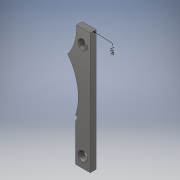
# Autodesk Inventor part: 1-4inch_FixedKnifeSmall_Piece1
Saved by Autodesk Inventor 2018 (Build 220112000, 112)
## iProperties
Created: 2018-01-21
Part Number: 1-4inch_FixedKnifeSmall_Piece1
Material: Generic
Document SubType Name: Modeling
Designer: Olivier
Density: 1 g/cm^3
Appearance: Default
Author: Olivier
Autodesk Inventor part; units mm, degrees
ref_plane "YZ Plane" through (0, 0, 0) normal (1, 0, 0) x (0, 1, 0)
ref_plane "XZ Plane" through (0, 0, 0) normal (0, 1, 0) x (-1, 0, 0)
ref_plane "XY Plane" through (0, 0, 0) normal (0, 0, 1) x (1, 0, 0)
sketch "Sketch1" plane through (0, 0, 0) normal (0, 0, 1) x (1, 0, 0)
  arc A0 (-24.5815, 32.7806) -> (-15, 60) centre (-62.8769, 61.5571) ccw
  arc A1 (-16.2637, 17.2484) -> (-24.5815, 32.7806) centre (-62.817, 2.3111) ccw
  arc A2 (-16, -20.3999) -> (-16.2637, 17.2484) centre (-70.52, -1.9566) ccw
  line L0 (-16, -20.3999) -> (-13.5, -21.5)
  line L1 (-13.5, -21.5) -> (-16, -25.9706)
  line L2 (-16, -25.9706) -> (-16, -67)
  line L3 (-16, -67) -> (0, -67)
  line L4 (0, -67) -> (0, 65)
  line L5 (0, 65) -> (-15, 65)
  line L6 (-15, 65) -> (-15, 60)
  circle A3 centre (-8, 50) radius 5.25
  circle A4 centre (-8, -55.4085) radius 5.25
  arc A5 (-24.5815, 32.7806) -> (-15, 60) centre (-62.8769, 61.5571) ccw
  arc A6 (-16.2637, 17.2484) -> (-24.5815, 32.7806) centre (-62.817, 2.3111) ccw
  arc A7 (-16, -20.3999) -> (-16.2637, 17.2484) centre (-70.52, -1.9566) ccw
  line L7 (-16, -20.3999) -> (-13.5, -21.5)
  line L8 (-13.5, -21.5) -> (-16, -25.9706)
  line L9 (-16, -25.9706) -> (-16, -67)
  line L10 (-16, -67) -> (0, -67)
  line L11 (0, -67) -> (0, 65)
  line L12 (0, 65) -> (-15, 65)
  line L13 (-15, 65) -> (-15, 60)
  circle A8 centre (-8, 50) radius 5.25
  circle A9 centre (-8, -55.4085) radius 5.25
  point P0 (0, 0)
  constraints: 28 end point, 12 point on circle, 10 centre point
extrude "Extrusion1" add sketch "Sketch1" along normal blind 6.35
body "Solid1"
